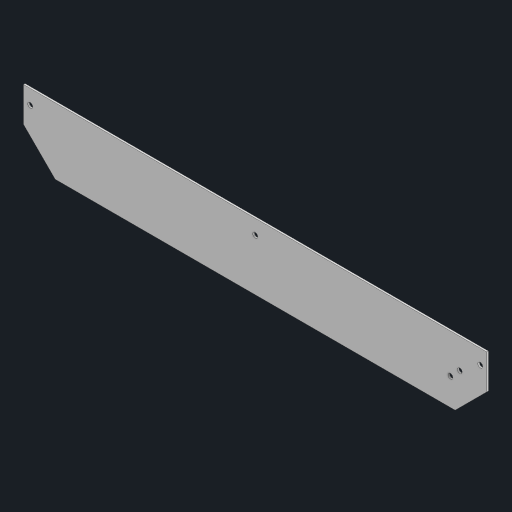
# Autodesk Inventor part: sideskirt
Saved by Autodesk Inventor 2023 (Build 270158000, 158)
## iProperties
Created: 2023-04-10
Part Number: sideskirt
Material: Generic
Document SubType Name: Modeling
Designer: Windows Macbook
Density: 1 g/cm^3
Appearance: Default
Author: Windows Macbook
Autodesk Inventor part; units mm, degrees
ref_plane "YZ Plane" through (0, 0, 0) normal (1, 0, 0) x (0, 1, 0)
ref_plane "XZ Plane" through (0, 0, 0) normal (0, 1, 0) x (-1, 0, 0)
ref_plane "XY Plane" through (0, 0, 0) normal (0, 0, 1) x (1, 0, 0)
sketch "Sketch1" plane through (0, 0, 0) normal (0, 0, 1) x (1, 0, 0)
  line L0 (444.5, 63.5) -> (0, 63.5)
  line L1 (0, 63.5) -> (0, 30.48)
  line L2 (0, 30.48) -> (30.48, 0)
  line L3 (30.48, 0) -> (414.02, 0)
  line L4 (444.5, 30.48) -> (444.5, 63.5)
  line L5 (0, 63.5) -> (0, 53.34)
  line L6 (444.5, 30.48) -> (414.02, 0)
  line L7 (444.5, 30.48) -> (487.6052, 30.48) construction
  point P0 (0, 0)
  dimension "d0" = 444.5
  dimension "d2" = 30.48
  dimension "d19" = 135
  constraints: 16 end point, 2 horizontal, 2 parallel, 1 equal length, 1 perpendicular, 1 point on line
  measures "d0" distance of L0.end L0.start
  measures "d2" distance of point (0, 0) L1.end
  measures "d19" angle of L6 L7
extrude "Extrusion1" add sketch "Sketch1" along normal blind 1.5875
sketch "Sketch2" plane through (0, 0, 1.5875) normal (0, 0, 1) x (1, 0, 0)
  line L0 (0.22, 63.5) -> (0.22, 50.8)
  line L1 (0.22, 50.8) -> (12.92, 63.5)
  line L2 (444.5, 63.5) -> (0, 63.5) projected
  line L3 (0, 63.5) -> (0, 30.48) projected
  line L4 (0, 63.5) -> (6.57, 57.15)
  line L5 (6.57, 57.15) -> (6.57, 49.53)
  line L6 (6.57, 57.15) -> (14.19, 57.15) construction
  line L7 (444.5, 30.48) -> (444.5, 63.5) projected
  line L8 (444.5, 63.5) -> (444.5, 50.8)
  line L9 (444.5, 50.8) -> (431.8, 63.5)
  line L10 (431.8, 63.5) -> (444.5, 63.5)
  line L11 (444.5, 63.5) -> (438.15, 57.15)
  line L12 (438.15, 57.15) -> (438.15, 49.53)
  line L13 (438.15, 49.53) -> (6.57, 49.53)
  line L14 (30.48, 0) -> (414.02, 0) projected
  line L15 (414.02, 0) -> (444.5, 30.48)
  line L16 (414.02, 0) -> (444.5, 30.48) projected
  line L17 (429.26, 15.24) -> (444.5, 0)
  line L18 (429.26, 15.24) -> (413.9711, 30.5289)
  line L19 (418.4613, 35.019) -> (409.481, 26.0387)
  line L20 (429.26, 15.24) -> (414.8916, 29.6084)
  point P0 (0, 0)
  point P1 (0, 30.48)
  point P2 (222.36, 49.53)
  point P3 (409.481, 26.0387)
  dimension "d9" = 12.7
  dimension "d10" = 45
  dimension "d20" = 7.62
  dimension "d21" = 90
  dimension "d22" = 12.7
  dimension "d23" = 45
  dimension "d24" = 7.62
  dimension "d33" = 6.35
  constraints: 32 end point, 6 point on line, 5 perpendicular, 4 coincident, 4 midpoint, 2 vertical, 1 collinear, 1 horizontal, 1 other
  measures "d9" distance of L0.start L0.end
  measures "d10" angle of L1 L0
  measures "d20" distance of L4.end L5.end
  measures "d21" angle of L5 L6
  measures "d22" distance of L2.start L8.end
  measures "d23" angle of L8 L9
  measures "d24" distance of L11.end L12.end
  measures "d33" distance of L18.end L19.start
hole "Hole2" at (6.57, 49.53, 1.5875) at (222.36, 49.53, 1.5875) at (438.15, 49.53, 1.5875) at (418.4613, 35.019, 1.5875) at (409.481, 26.0387, 1.5875) direction (0, 0, -1) diameter 4.7625 end through all
body "Solid1"
